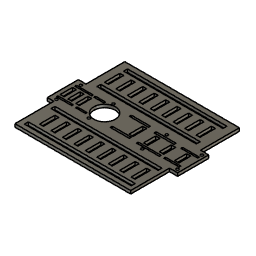
Drone Platform v10 - Top Layer (Autodesk Fusion 360 design; units mm, degrees)
Autodesk Fusion 360 part; units mm, degrees
sketch "Sketch1" plane through (0, 0, 0) normal (0, 0, 1) x (1, 0, 0)
  line L0 (0, 40.6706) -> (170.6716, 40.6706)
  line L1 (170.6716, 40.6706) -> (170.6716, 0)
  line L2 (170.6716, 0) -> (0, 0)
  line L3 (0, 0) -> (0, 40.6706)
  constraint horizontal L0
  constraint vertical L1
  constraint horizontal L2
  constraint vertical L3
sketch "Sketch2" plane through (0, 0, 0) normal (0, 0, 1) x (1, 0, 0)
  circle A0 centre (2.5, 4) radius 1.75
  line L0 (170.6716, 0) -> (0, 0)
  line L1 (0, 0) -> (0, 40.6706)
  dimension "d1" = 3.5
  dimension "d2" = 4
  dimension "d3" = 2.5
  measures "d1" diameter of A0
  measures "d2" distance of A0.centre L0
  measures "d3" distance of A0.centre L1
sketch "Sketch4" plane through (0, 0, 0) normal (0, 0, 1) x (1, 0, 0)
  circle A0 centre (49.5, 4) radius 1.75
  circle A1 centre (2.5, 4) radius 1.75
  dimension "d9" = 3.5
  dimension "d10" = 47
  measures "d9" diameter of A0
  measures "d10" distance of A0.centre A1.centre
extrude "Extrude1" add sketch "Sketch1" along normal blind 4
sketch "Sketch11" plane through (0, 0, 4) normal (0, 0, 1) x (-1, 0, 0)
  line L0 (0, 0) -> (-170.6716, 0)
  line L1 (-170.6716, 0) -> (-170.6716, -40.6706)
  line L2 (-170.6716, -40.6706) -> (0, -40.6706)
  line L3 (0, -40.6706) -> (0, 0)
  line L4 (-5, -30) -> (-150, -30)
  line L5 (-150, -30) -> (-150, -10)
  line L6 (-150, -10) -> (-5, -10)
  line L7 (-5, -10) -> (-5, -30)
  constraint horizontal L4
  constraint vertical L5
  constraint horizontal L6
  constraint vertical L7
sketch "Sketch13" plane through (0, 0, 4) normal (0, 0, 1) x (-1, 0, 0)
  line L0 (0, 0) -> (-170.6716, 0)
  line L1 (-170.6716, 0) -> (-170.6716, -40.6706)
  line L2 (-170.6716, -40.6706) -> (0, -40.6706)
  line L3 (0, -40.6706) -> (0, 0)
  circle A0 centre (-8, -4) radius 1.75
  circle A1 centre (-8, -36) radius 1.75
  circle A2 centre (-50.5, -36) radius 1.75
  circle A3 centre (-50.5, -4) radius 1.75
  circle A4 centre (-120.5, -4) radius 1.75
  circle A5 centre (-120.5, -36) radius 1.75
  circle A6 centre (-166.5, -4) radius 1.75
  circle A7 centre (-166.5, -36) radius 1.75
  dimension "d44" = 3.5
  dimension "d45" = 4
  dimension "d46" = 3.5
  dimension "d47" = 32
  dimension "d48" = 8
  dimension "d49" = 8
  dimension "d50" = 3.5
  dimension "d52" = 3.5
  dimension "d53" = 4
  dimension "d55" = 32
  dimension "d56" = 3.5
  dimension "d58" = 4
  dimension "d59" = 3.5
  dimension "d60" = 32
  dimension "d62" = 3.5
  dimension "d63" = 46
  dimension "d64" = 4
  dimension "d65" = 3.5
  dimension "d66" = 46
  dimension "d67" = 32
  measures "d44" diameter of A0
  measures "d45" distance of L0 A0.centre
  measures "d46" diameter of A1
  measures "d47" vertical distance of A0.centre A1.centre
  measures "d48" distance of L3 A1.centre
  measures "d49" distance of L3 A0.centre
  measures "d50" diameter of A2
  measures "d52" diameter of A3
  measures "d53" distance of L0 A3.centre
  measures "d55" distance of A2.centre A3.centre
  measures "d56" diameter of A4
  measures "d58" distance of L0 A4.centre
  measures "d59" diameter of A5
  measures "d60" distance of A4.centre A5.centre
  measures "d62" diameter of A6
  measures "d63" distance of A4.centre A6.centre
  measures "d64" distance of L0 A6.centre
  measures "d65" diameter of A7
  measures "d66" horizontal distance of A5.centre A7.centre
  measures "d67" distance of A6.centre A7.centre
extrude "Extrude5" cut sketch "Sketch13" against normal blind 15 contours A0 | A1 | A2 | A3 | A4 | A5 | A6 | A7
sketch "Sketch16" plane through (0, 0, 4) normal (0, 0, 1) x (-1, 0, 0)
  circle A0 centre (-120.5, -36) radius 1.75
  circle A1 centre (-50.5, -36) radius 1.75
  circle A2 centre (-50.5, -4) radius 1.75
  circle A3 centre (-120.5, -4) radius 1.75
  circle A4 centre (-166.5, -36) radius 1.75
  circle A5 centre (-8, -36) radius 1.75
  circle A6 centre (-8, -4) radius 1.75
  circle A7 centre (-166.5, -4) radius 1.75
  line L0 (0, 0) -> (-170.6716, 0)
  line L1 (-170.6716, 0) -> (-170.6716, -40.6706)
  line L2 (-170.6716, -40.6706) -> (0, -40.6706)
  line L3 (0, -40.6706) -> (0, 0)
  line L4 (-5, -33) -> (-27, -33)
  line L5 (-27, -33) -> (-27, -31)
  line L6 (-27, -31) -> (-5, -31)
  line L7 (-5, -31) -> (-5, -33)
  line L8 (-5, -6.9037) -> (-25, -6.9037)
  line L9 (-25, -6.9037) -> (-25, -8.99)
  line L10 (-25, -8.99) -> (-5, -8.99)
  line L11 (-5, -8.99) -> (-5, -6.9037)
  line L12 (-5, -28.024) -> (-10, -28.024)
  line L13 (-10, -28.024) -> (-10, -12)
  line L14 (-10, -12) -> (-5, -12)
  line L15 (-5, -12) -> (-5, -28.024)
  line L16 (-15, -28) -> (-20, -28)
  line L17 (-20, -28) -> (-20, -12)
  line L18 (-20, -12) -> (-15, -12)
  line L19 (-15, -12) -> (-15, -28)
  line L20 (-25.2942, -28) -> (-30, -28)
  line L21 (-30, -28) -> (-30, -12)
  line L22 (-30, -12) -> (-25.2942, -12)
  line L23 (-25.2942, -12) -> (-25.2942, -28)
  line L24 (-30, -33) -> (-43, -33)
  line L25 (-43, -33) -> (-43, -31)
  line L26 (-43, -31) -> (-30, -31)
  line L27 (-30, -31) -> (-30, -33)
  line L28 (-30, -9) -> (-43, -9)
  line L29 (-43, -9) -> (-43, -7)
  line L30 (-43, -7) -> (-30, -7)
  line L31 (-30, -7) -> (-30, -9)
  circle A8 centre (-55, -20) radius 14.1421
  line L32 (-94.9908, -12) -> (-100.1485, -12)
  line L33 (-100.1485, -12) -> (-100.1485, -30)
  line L34 (-100.1485, -30) -> (-94.9908, -30)
  line L35 (-94.9908, -30) -> (-94.9908, -12)
  line L36 (-114.4734, -27.5201) -> (-119.9683, -27.5201)
  line L37 (-119.9683, -27.5201) -> (-119.9683, -11.6326)
  line L38 (-119.9683, -11.6326) -> (-114.4734, -11.6326)
  line L39 (-114.4734, -11.6326) -> (-114.4734, -27.5201)
  line L40 (-134.7975, -27.5201) -> (-140.4499, -27.5201)
  line L41 (-140.4499, -27.5201) -> (-140.4499, -12)
  line L42 (-140.4499, -12) -> (-134.7975, -12)
  line L43 (-134.7975, -12) -> (-134.7975, -27.5201)
  line L44 (-154.7885, -27.5201) -> (-160.2653, -27.5201)
  line L45 (-160.2653, -27.5201) -> (-160.2653, -12)
  line L46 (-160.2653, -12) -> (-154.7885, -12)
  line L47 (-154.7885, -12) -> (-154.7885, -27.5201)
  line L48 (-75, -10) -> (-100, -10)
  line L49 (-100, -10) -> (-100, -7.452)
  line L50 (-100, -7.452) -> (-75, -7.452)
  line L51 (-75, -7.452) -> (-75, -10)
  line L52 (-110, -8.9897) -> (-139.8992, -8.9897)
  line L53 (-139.8992, -8.9897) -> (-139.8992, -6.7652)
  line L54 (-139.8992, -6.7652) -> (-110, -6.7652)
  line L55 (-110, -6.7652) -> (-110, -8.9897)
  line L56 (-145, -9.7245) -> (-165.0971, -9.7245)
  line L57 (-165.0971, -9.7245) -> (-165.0971, -7.5785)
  line L58 (-165.0971, -7.5785) -> (-145, -7.5785)
  line L59 (-145, -7.5785) -> (-145, -9.7245)
  line L60 (-75, -35) -> (-99.8075, -35)
  line L61 (-99.8075, -35) -> (-99.8075, -32.5523)
  line L62 (-99.8075, -32.5523) -> (-75, -32.5523)
  line L63 (-75, -32.5523) -> (-75, -35)
  line L64 (-110, -32.4558) -> (-136, -32.4558)
  line L65 (-136, -32.4558) -> (-136, -29.8985)
  line L66 (-136, -29.8985) -> (-110, -29.8985)
  line L67 (-110, -29.8985) -> (-110, -32.4558)
  line L68 (-145, -31.9897) -> (-167, -31.9897)
  line L69 (-167, -31.9897) -> (-167, -29.9185)
  line L70 (-167, -29.9185) -> (-145, -29.9185)
  line L71 (-145, -29.9185) -> (-145, -31.9897)
  dimension "d78" = 22
  dimension "d79" = 3
  dimension "d81" = 13
  dimension "d82" = 13
  constraint horizontal L4
  constraint vertical L5
  constraint horizontal L6
  constraint vertical L7
  constraint horizontal L8
  constraint vertical L9
  constraint horizontal L10
  constraint vertical L11
  constraint horizontal L12
  constraint vertical L13
  constraint horizontal L14
  constraint vertical L15
  constraint horizontal L16
  constraint vertical L17
  constraint horizontal L18
  constraint vertical L19
  constraint horizontal L20
  constraint vertical L21
  constraint horizontal L22
  constraint vertical L23
  constraint horizontal L24
  constraint vertical L25
  constraint horizontal L26
  constraint vertical L27
  constraint horizontal L28
  constraint vertical L29
  constraint horizontal L30
  constraint vertical L31
  constraint horizontal L32
  constraint vertical L33
  constraint horizontal L34
  constraint vertical L35
  constraint horizontal L36
  constraint vertical L37
  constraint horizontal L38
  constraint vertical L39
  constraint horizontal L40
  constraint vertical L41
  constraint horizontal L42
  constraint vertical L43
  constraint horizontal L44
  constraint vertical L45
  constraint horizontal L46
  constraint vertical L47
  constraint horizontal L48
  constraint vertical L49
  constraint horizontal L50
  constraint vertical L51
  constraint horizontal L52
  constraint vertical L53
  constraint horizontal L54
  constraint vertical L55
  constraint horizontal L56
  constraint vertical L57
  constraint horizontal L58
  constraint vertical L59
  constraint horizontal L60
  constraint vertical L61
  constraint horizontal L62
  constraint vertical L63
  constraint horizontal L64
  constraint vertical L65
  constraint horizontal L66
  constraint vertical L67
  constraint horizontal L68
  constraint vertical L69
  constraint horizontal L70
  constraint vertical L71
  measures "d78" distance of L4.start L4.end
  measures "d79" distance of L5 L27
  measures "d81" distance of L24.start L24.end
  measures "d82" distance of L28.start L28.end
extrude "Extrude8" cut sketch "Sketch16" against normal blind 15 contours L4 L5 L6 L7 | L8 L9 L10 L11 | L12 L13 L14 L15 | L16 L17 L18 L19 | L20 L21 L22 L23 | L24 L25 L26 L27 | L28 L29 L30 L31 | A8 | L32 L33 L34 L35 | L36 L37 L38 L39 | L40 L41 L42 L43 | L44 L45 L46 L47 | L48 L49 L50 L51 | L52 L53 L54 L55 | L56 L57 L58 L59 | L60 L61 L62 L63 | L64 L65 L66 L67 | L68 L69 L70 L71
sketch "Sketch17" plane through (0, 0, 0) normal (0, -1, 0) x (1, 0, 0)
  line L0 (0, 0) -> (170.6716, 0)
  line L1 (170.6716, 0) -> (170.6716, 4)
  line L2 (170.6716, 4) -> (0, 4)
  line L3 (0, 4) -> (0, 0)
  line L4 (8.4404, 4) -> (160, 4)
  line L5 (160, 4) -> (160, 0)
  line L6 (160, 0) -> (8.4404, 0)
  line L7 (8.4404, 0) -> (8.4404, 4)
  constraint horizontal L4
  constraint vertical L5
  constraint horizontal L6
  constraint vertical L7
  constraint coincident L0 L5.end
  constraint coincident L2 L4.start
extrude "Extrude9" add sketch "Sketch17" along normal blind 50.8 contours L0 L2 L4 L5 L6 L7
sketch "Sketch18" plane through (0, 40.6706, 0) normal (0, 1, 0) x (-1, 0, 0)
  line L0 (-170.6716, 0) -> (0, 0)
  line L1 (0, 0) -> (0, 4)
  line L2 (0, 4) -> (-170.6716, 4)
  line L3 (-170.6716, 4) -> (-170.6716, 0)
  line L4 (-160.0228, 4) -> (-10, 4)
  line L5 (-10, 4) -> (-10, 0)
  line L6 (-10, 0) -> (-160.0228, 0)
  line L7 (-160.0228, 0) -> (-160.0228, 4)
  constraint horizontal L4
  constraint vertical L5
  constraint horizontal L6
  constraint vertical L7
  constraint coincident L0 L5.end
  constraint coincident L2 L4.start
extrude "Extrude10" add sketch "Sketch18" along normal blind 50.8 contours L0 L2 L4 L5 L6 L7
sketch "Sketch19" plane through (0, 0, 4) normal (0, 0, 1) x (-1, 0, 0)
  line L0 (-167, -31.9897) -> (-167, -29.9185)
  line L1 (-167, -29.9185) -> (-145, -29.9185)
  line L2 (-145, -29.9185) -> (-145, -31.9897)
  line L3 (-145, -31.9897) -> (-167, -31.9897)
  line L4 (-136, -32.4558) -> (-136, -29.8985)
  line L5 (-136, -29.8985) -> (-110, -29.8985)
  line L6 (-110, -29.8985) -> (-110, -32.4558)
  line L7 (-110, -32.4558) -> (-136, -32.4558)
  line L8 (-43, -9) -> (-43, -7)
  line L9 (-43, -7) -> (-30, -7)
  line L10 (-30, -7) -> (-30, -9)
  line L11 (-30, -9) -> (-43, -9)
  line L12 (-30, -28) -> (-30, -12)
  line L13 (-30, -12) -> (-25.2942, -12)
  line L14 (-25.2942, -12) -> (-25.2942, -28)
  line L15 (-25.2942, -28) -> (-30, -28)
  circle A0 centre (-55, -20) radius 14.1421
  line L16 (-20, -28) -> (-20, -12)
  line L17 (-20, -12) -> (-15, -12)
  line L18 (-15, -12) -> (-15, -28)
  line L19 (-15, -28) -> (-20, -28)
  line L20 (-100, -10) -> (-100, -7.452)
  line L21 (-100, -7.452) -> (-75, -7.452)
  line L22 (-75, -7.452) -> (-75, -10)
  line L23 (-75, -10) -> (-100, -10)
  line L24 (-140.4499, -27.5201) -> (-140.4499, -12)
  line L25 (-140.4499, -12) -> (-134.7975, -12)
  line L26 (-134.7975, -12) -> (-134.7975, -27.5201)
  line L27 (-134.7975, -27.5201) -> (-140.4499, -27.5201)
  line L28 (-160.2653, -27.5201) -> (-160.2653, -12)
  line L29 (-160.2653, -12) -> (-154.7885, -12)
  line L30 (-154.7885, -12) -> (-154.7885, -27.5201)
  line L31 (-154.7885, -27.5201) -> (-160.2653, -27.5201)
  line L32 (-139.8992, -8.9897) -> (-139.8992, -6.7652)
  line L33 (-139.8992, -6.7652) -> (-110, -6.7652)
  line L34 (-110, -6.7652) -> (-110, -8.9897)
  line L35 (-110, -8.9897) -> (-139.8992, -8.9897)
  line L36 (-99.8075, -35) -> (-99.8075, -32.5523)
  line L37 (-99.8075, -32.5523) -> (-75, -32.5523)
  line L38 (-75, -32.5523) -> (-75, -35)
  line L39 (-75, -35) -> (-99.8075, -35)
  line L40 (-25, -6.9037) -> (-5, -6.9037)
  line L41 (-5, -6.9037) -> (-5, -8.99)
  line L42 (-5, -8.99) -> (-25, -8.99)
  line L43 (-25, -8.99) -> (-25, -6.9037)
  line L44 (-43, -33) -> (-43, -31)
  line L45 (-43, -31) -> (-30, -31)
  line L46 (-30, -31) -> (-30, -33)
  line L47 (-30, -33) -> (-43, -33)
  line L48 (-27, -33) -> (-27, -31)
  line L49 (-27, -31) -> (-5, -31)
  line L50 (-5, -31) -> (-5, -33)
  line L51 (-5, -33) -> (-27, -33)
  line L52 (-10, -28.024) -> (-10, -12)
  line L53 (-10, -12) -> (-5, -12)
  line L54 (-5, -12) -> (-5, -28.024)
  line L55 (-5, -28.024) -> (-10, -28.024)
  line L56 (-100.1485, -12) -> (-94.9908, -12)
  line L57 (-94.9908, -12) -> (-94.9908, -30)
  line L58 (-94.9908, -30) -> (-100.1485, -30)
  line L59 (-100.1485, -30) -> (-100.1485, -12)
  line L60 (-119.9683, -27.5201) -> (-119.9683, -11.6326)
  line L61 (-119.9683, -11.6326) -> (-114.4734, -11.6326)
  line L62 (-114.4734, -11.6326) -> (-114.4734, -27.5201)
  line L63 (-114.4734, -27.5201) -> (-119.9683, -27.5201)
  line L64 (-165.0971, -9.7245) -> (-165.0971, -7.5785)
  line L65 (-165.0971, -7.5785) -> (-145, -7.5785)
  line L66 (-145, -7.5785) -> (-145, -9.7245)
  line L67 (-145, -9.7245) -> (-165.0971, -9.7245)
  circle A1 centre (-120.5, -36) radius 1.75
  circle A2 centre (-50.5, -36) radius 1.75
  circle A3 centre (-50.5, -4) radius 1.75
  circle A4 centre (-120.5, -4) radius 1.75
  circle A5 centre (-166.5, -36) radius 1.75
  circle A6 centre (-8, -36) radius 1.75
  circle A7 centre (-8, -4) radius 1.75
  circle A8 centre (-166.5, -4) radius 1.75
  line L68 (0, 0) -> (-8.4404, 0)
  line L69 (-8.4404, 0) -> (-8.4404, 50.8)
  line L70 (-8.4404, 50.8) -> (-160, 50.8)
  line L71 (-160, 50.8) -> (-160, 0)
  line L72 (-160, 0) -> (-170.6716, 0)
  line L73 (-170.6716, 0) -> (-170.6716, -40.6706)
  line L74 (-170.6716, -40.6706) -> (-160.0228, -40.6706)
  line L75 (-160.0228, -40.6706) -> (-160.0228, -91.4706)
  line L76 (-160.0228, -91.4706) -> (-10, -91.4706)
  line L77 (-10, -91.4706) -> (-10, -40.6706)
  line L78 (-10, -40.6706) -> (0, -40.6706)
  line L79 (0, -40.6706) -> (0, 0)
  line L80 (-155, 45) -> (-15.1018, 45)
  line L81 (-15.1018, 45) -> (-15.1018, 40)
  line L82 (-15.1018, 40) -> (-155, 40)
  line L83 (-155, 40) -> (-155, 45)
  line L84 (-155, 10) -> (-15, 10)
  line L85 (-15, 10) -> (-15, 5)
  line L86 (-15, 5) -> (-155, 5)
  line L87 (-155, 5) -> (-155, 10)
  line L88 (-150, 35) -> (-145, 35)
  line L89 (-145, 35) -> (-145, 15)
  line L90 (-145, 15) -> (-150, 15)
  line L91 (-150, 15) -> (-150, 35)
  line L92 (-135, 35) -> (-130, 35)
  line L93 (-130, 35) -> (-130, 15)
  line L94 (-130, 15) -> (-135, 15)
  line L95 (-135, 15) -> (-135, 35)
  line L96 (-120, 35) -> (-115, 35)
  line L97 (-115, 35) -> (-115, 15)
  line L98 (-115, 15) -> (-120, 15)
  line L99 (-120, 15) -> (-120, 35)
  line L100 (-105, 35) -> (-100, 35)
  line L101 (-100, 35) -> (-100, 15)
  line L102 (-100, 15) -> (-105, 15)
  line L103 (-105, 15) -> (-105, 35)
  line L104 (-90, 35) -> (-85, 35)
  line L105 (-85, 35) -> (-85, 15)
  line L106 (-85, 15) -> (-90, 15)
  line L107 (-90, 15) -> (-90, 35)
  line L108 (-75, 35) -> (-70, 35)
  line L109 (-70, 35) -> (-70, 15)
  line L110 (-70, 15) -> (-75, 15)
  line L111 (-75, 15) -> (-75, 35)
  line L112 (-60, 35) -> (-55, 35)
  line L113 (-55, 35) -> (-55, 15)
  line L114 (-55, 15) -> (-60, 15)
  line L115 (-60, 15) -> (-60, 35)
  line L116 (-45, 35) -> (-40, 35)
  line L117 (-40, 35) -> (-40, 15)
  line L118 (-40, 15) -> (-45, 15)
  line L119 (-45, 15) -> (-45, 35)
  line L120 (-30, 35) -> (-25, 35)
  line L121 (-25, 35) -> (-25, 15)
  line L122 (-25, 15) -> (-30, 15)
  line L123 (-30, 15) -> (-30, 35)
  line L124 (-150, -80) -> (-20, -80)
  line L125 (-20, -80) -> (-20, -85)
  line L126 (-20, -85) -> (-150, -85)
  line L127 (-150, -85) -> (-150, -80)
  line L128 (-150, -45) -> (-20, -45)
  line L129 (-20, -45) -> (-20, -50)
  line L130 (-20, -50) -> (-150, -50)
  line L131 (-150, -50) -> (-150, -45)
  line L132 (-145, -55) -> (-140, -55)
  line L133 (-140, -55) -> (-140, -75)
  line L134 (-140, -75) -> (-145, -75)
  line L135 (-145, -75) -> (-145, -55)
  line L136 (-130, -55) -> (-125, -55)
  line L137 (-125, -55) -> (-125, -75)
  line L138 (-125, -75) -> (-130, -75)
  line L139 (-130, -75) -> (-130, -55)
  line L140 (-115, -55) -> (-110, -55)
  line L141 (-110, -55) -> (-110, -75)
  line L142 (-110, -75) -> (-115, -75)
  line L143 (-115, -75) -> (-115, -55)
  line L144 (-100, -55) -> (-95, -55)
  line L145 (-95, -55) -> (-95, -75)
  line L146 (-95, -75) -> (-100, -75)
  line L147 (-100, -75) -> (-100, -55)
  line L148 (-85, -55) -> (-80, -55)
  line L149 (-80, -55) -> (-80, -75)
  line L150 (-80, -75) -> (-85, -75)
  line L151 (-85, -75) -> (-85, -55)
  line L152 (-70, -55) -> (-65, -55)
  line L153 (-65, -55) -> (-65, -75)
  line L154 (-65, -75) -> (-70, -75)
  line L155 (-70, -75) -> (-70, -55)
  line L156 (-55, -55) -> (-50, -55)
  line L157 (-50, -55) -> (-50, -75)
  line L158 (-50, -75) -> (-55, -75)
  line L159 (-55, -75) -> (-55, -55)
  line L160 (-40, -55) -> (-35, -55)
  line L161 (-35, -55) -> (-35, -75)
  line L162 (-35, -75) -> (-40, -75)
  line L163 (-40, -75) -> (-40, -55)
  line L164 (-25, -55) -> (-20, -55)
  line L165 (-20, -55) -> (-20, -75)
  line L166 (-20, -75) -> (-25, -75)
  line L167 (-25, -75) -> (-25, -55)
  constraint horizontal L80
  constraint vertical L81
  constraint horizontal L82
  constraint vertical L83
  constraint horizontal L84
  constraint vertical L85
  constraint horizontal L86
  constraint vertical L87
  constraint horizontal L88
  constraint vertical L89
  constraint horizontal L90
  constraint vertical L91
  constraint horizontal L92
  constraint vertical L93
  constraint horizontal L94
  constraint vertical L95
  constraint horizontal L96
  constraint vertical L97
  constraint horizontal L98
  constraint vertical L99
  constraint horizontal L100
  constraint vertical L101
  constraint horizontal L102
  constraint vertical L103
  constraint horizontal L104
  constraint vertical L105
  constraint horizontal L106
  constraint vertical L107
  constraint horizontal L108
  constraint vertical L109
  constraint horizontal L110
  constraint vertical L111
  constraint horizontal L112
  constraint vertical L113
  constraint horizontal L114
  constraint vertical L115
  constraint horizontal L116
  constraint vertical L117
  constraint horizontal L118
  constraint vertical L119
  constraint horizontal L120
  constraint vertical L121
  constraint horizontal L122
  constraint vertical L123
  constraint horizontal L124
  constraint vertical L125
  constraint horizontal L126
  constraint vertical L127
  constraint horizontal L128
  constraint vertical L129
  constraint horizontal L130
  constraint vertical L131
  constraint horizontal L132
  constraint vertical L133
  constraint horizontal L134
  constraint vertical L135
  constraint horizontal L136
  constraint vertical L137
  constraint horizontal L138
  constraint vertical L139
  constraint horizontal L140
  constraint vertical L141
  constraint horizontal L142
  constraint vertical L143
  constraint horizontal L144
  constraint vertical L145
  constraint horizontal L146
  constraint vertical L147
  constraint horizontal L148
  constraint vertical L149
  constraint horizontal L150
  constraint vertical L151
  constraint horizontal L152
  constraint vertical L153
  constraint horizontal L154
  constraint vertical L155
  constraint horizontal L156
  constraint vertical L157
  constraint horizontal L158
  constraint vertical L159
  constraint horizontal L160
  constraint vertical L161
  constraint horizontal L162
  constraint vertical L163
  constraint horizontal L164
  constraint vertical L165
  constraint horizontal L166
  constraint vertical L167
extrude "Extrude11" cut sketch "Sketch19" against normal blind 20 contours L80 L81 L82 L83 | L84 L85 L86 L87 | L88 L89 L90 L91 | L92 L93 L94 L95 | L96 L97 L98 L99 | L100 L101 L102 L103 | L104 L105 L106 L107 | L108 L109 L110 L111 | L112 L113 L114 L115 | L116 L117 L118 L119 | L120 L121 L122 L123 | L124 L125 L126 L127 | L128 L129 L130 L131 | L132 L133 L134 L135 | L136 L137 L138 L139 | L140 L141 L142 L143 | L144 L145 L146 L147 | L148 L149 L150 L151 | L152 L153 L154 L155 | L156 L157 L158 L159 | L160 L161 L162 L163 | L164 L165 L166 L167
